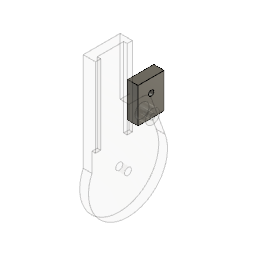
single slider crank v2 (Autodesk Fusion 360 design; units mm, degrees)
Autodesk Fusion 360 part; units mm, degrees
sketch "Sketch1" plane through (0, 0, 0) normal (1, 0, 0) x (0, 1, 0) in component "c1"
  circle A0 centre (0, 0) radius 4
  line L0 (-40.9987, 18.55) -> (-40.9987, 130.55)
  line L1 (-40.9987, 130.55) -> (1.0013, 130.55)
  line L2 (1.0013, 130.55) -> (1.0013, 65.55)
  line L3 (1.0013, 65.55) -> (17.0013, 65.55)
  arc A1 (26.8331, 53.724) -> (17.0013, 65.55) centre (17.0013, 55.55) ccw
  line L4 (26.3963, 58.9752) -> (42.2779, 15.4135)
  circle A2 centre (16, 52) radius 8
  circle A3 centre (16, 52) radius 3
  arc A4 (-40.9987, 18.55) -> (42.2779, 15.4135) centre (0, 0) ccw
  dimension "d1" = 90
  dimension "d2" = 8
  dimension "d3" = 112
  dimension "d4" = 18.55
  dimension "d5" = 42
  dimension "d6" = 65
  dimension "d7" = 16
  dimension "d9" = 10
  dimension "d10" = 16
  dimension "d11" = 6
  dimension "d12" = 52
  dimension "d13" = 16
  constraint coincident A0.centre A4.centre
  constraint concentric A0 A4
  constraint vertical L0
  constraint perpendicular L0 L1
  constraint perpendicular L1 L2
  constraint perpendicular L2 L3
  constraint tangent L3 A1
  constraint coincident A1 L4.start
  constraint tangent A1 L4
  constraint tangent L4 A4
  constraint concentric A2 A3
  measures "d1" diameter of A4
  measures "d2" diameter of A0
  measures "d3" distance of L0.start L0.end
  measures "d4" vertical distance of A0.centre L0.start
  measures "d5" distance of L0.end L1.end
  measures "d6" distance of L1.end L2.end
  measures "d7" distance of L2.end L3.end
  measures "d9" radius of A1
  measures "d10" diameter of A2
  measures "d11" diameter of A3
  measures "d12" vertical distance of A0.centre A2.centre
  measures "d13" horizontal distance of A0.centre A2.centre
extrude "Extrude1" add sketch "Sketch1" along normal blind 10 contours L0 L1 L2 L3 A1 L4 A4 makes body 1 in component "c1"
extrude "Extrude2" add sketch "Sketch1" along normal blind 22 contours A2 bodies 1 in component "c1"
sketch "Sketch2" plane through (10, 0, 0) normal (1, 0, 0) x (0, 1, 0) in component "c1"
  circle A0 centre (16, 52) radius 8
  circle A1 centre (0, 0) radius 4
  line L0 (-40.9987, 130.55) -> (-40.9987, 18.55)
  arc A2 (-40.9987, 18.55) -> (42.2779, 15.4135) centre (0, 0) ccw
  line L1 (42.2779, 15.4135) -> (26.3963, 58.9752)
  arc A3 (26.3963, 58.9752) -> (17.0013, 65.55) centre (17.0013, 55.55) ccw
  line L2 (17.0013, 65.55) -> (1.0013, 65.55)
  line L3 (1.0013, 65.55) -> (1.0013, 130.55)
  line L4 (1.0013, 130.55) -> (-40.9987, 130.55)
  line L5 (-40.9987, 130.55) -> (-34.9987, 130.55)
  line L6 (-34.9987, 130.55) -> (-34.9987, 40.4114)
  line L7 (-34.9987, 40.4114) -> (-40.9987, 40.4114)
  line L8 (-40.9987, 40.4114) -> (-40.9987, 130.55)
  line L9 (1.0013, 130.55) -> (-4.9987, 130.55)
  line L10 (-4.9987, 130.55) -> (-4.9987, 40.4114)
  line L11 (-4.9987, 40.4114) -> (1.0013, 40.4114)
  line L12 (1.0013, 40.4114) -> (1.0013, 130.55)
  dimension "d18" = 6
  dimension "d19" = 6
  constraint horizontal L5
  constraint vertical L6
  constraint horizontal L7
  constraint vertical L8
  constraint coincident L0.start L4.end
  constraint horizontal L9
  constraint vertical L10
  constraint horizontal L11
  constraint vertical L12
  constraint coincident L3.end L4.start
  measures "d18" distance of L0.start L5.end
  measures "d19" distance of L3.end L9.end
extrude "Extrude3" add sketch "Sketch2" along normal blind 4 contours L0 L4 L5 L6 L7 L8 | L3 L4 L9 L10 L11 L12 bodies 1 in component "c1"
sketch "Sketch1 (2)" plane through (0, 0, 0) normal (1, 0, 0) x (0, 1, 0) in component "c2"
  line L0 (0, 0) -> (30, 0)
  line L1 (30, 0) -> (30, 40)
  line L2 (30, 40) -> (0, 40)
  line L3 (0, 40) -> (0, 0)
  circle A0 centre (15, 25) radius 3
  dimension "d31" = 30
  dimension "d32" = 40
  dimension "d33" = 6
  dimension "d34" = 15
  dimension "d35" = 25
  constraint horizontal L0
  constraint vertical L1
  constraint horizontal L2
  constraint vertical L3
  constraint coincident L0.start L3.end
  measures "d31" distance of L0.start L0.end
  measures "d32" distance of L0.start L2.end
  measures "d33" diameter of A0
  measures "d34" distance of L3 A0.centre
  measures "d35" distance of L0 A0.centre
extrude "Extrude1'" add sketch "Sketch1 (2)" along normal blind 12 separate body makes body 2 in component "c2"
sketch "Sketch2 (2)" plane through (0, 0, 0) normal (1, 0, 0) x (0, 1, 0) in component "c2"
component "c1" placed x (1, 0, 0) y (0, 1, 0) z (0, 0, 1) at (0, 0, 0)
component "c2" placed x (-1, 0, 0) y (0, -1, 0) z (0, 0, 1) at (10, 41.3963, 38.9752)
